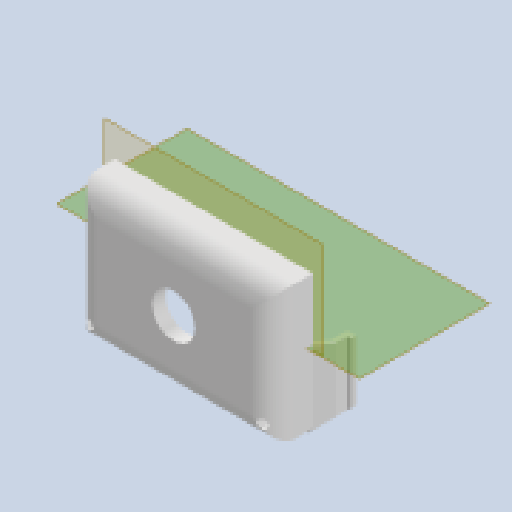
# Autodesk Inventor part: крышка камера
Saved by Autodesk Inventor 2024.2 (Build 282272000, 272)
## iProperties
Created: 2025-10-05
Part Number: крышка камера
Material: Типовые
Document SubType Name: Modeling
Designer: katya_notebook
Density: 1 g/cm^3
Appearance: По умолчанию
Author: katya_notebook
Autodesk Inventor part; units mm, degrees
ref_plane "YZ Plane" through (0, 0, 0) normal (1, 0, 0) x (0, 1, 0)
ref_plane "XZ Plane" through (0, 0, 0) normal (0, 1, 0) x (-1, 0, 0)
ref_plane "XY Plane" through (0, 0, 0) normal (0, 0, 1) x (1, 0, 0)
ref_plane "РабПлоскость1" through (0, 0, 0) normal (0, 0, 1) x (1, 0, 0)
sketch "Эскиз1" plane through (0, 0, 0) normal (0, 0, 1) x (1, 0, 0)
  line L0 (73.8991, -26.68) -> (-0.5009, -26.68) projected
  line L1 (53.6991, 17.5343) -> (19.6991, 17.5343) projected
  line L2 (0, 17.5343) -> (0, -26.68)
  line L3 (0, -26.68) -> (73.3991, -26.68)
  line L4 (73.3991, -13.5) -> (73.3991, 13.5) projected
  line L5 (73.3991, 17.5343) -> (73.3991, -26.68)
  line L6 (0, 17.5343) -> (0, 23.0229)
  line L7 (73.3991, 17.5343) -> (73.3991, 23.0229)
  line L8 (73.3991, 23.0229) -> (0, 23.0229)
  constraints: 12 end point, 3 perpendicular, 1 horizontal, 1 point on line, 1 vertical
extrude "Выдавливание1" add sketch "Эскиз1" along normal blind 15
sketch "Эскиз2" plane through (0, 0, 0) normal (0, 0, -1) x (-1, 0, 0)
  point P0 (0, 0)
sketch "Эскиз3" plane through (0, 0, 0) normal (0, 0, 1) x (1, 0, 0)
  circle A0 centre (36.6991, -1.4657) radius 8 projected
  line L0 (53.6991, 17.5343) -> (19.6991, 17.5343) projected
  line L1 (19.6991, -20.4657) -> (53.6991, -20.4657) projected
  line L2 (17.6991, 15.5343) -> (17.6991, -18.4657) projected
  line L3 (55.6991, -18.4657) -> (55.6991, 15.5343) projected
  line L4 (57.6991, 19.5343) -> (15.6991, 19.5343)
  line L5 (15.6991, 19.5343) -> (15.6991, -22.4657)
  line L6 (15.6991, -22.4657) -> (57.6991, -22.4657)
  line L7 (57.6991, -22.4657) -> (57.6991, 19.5343)
  line L8 (57.6991, 19.5343) -> (15.6991, -22.4657) construction
  line L9 (15.6991, 19.5343) -> (57.6991, -22.4657) construction
  point P0 (0, 0)
  dimension "d2" = 42
  dimension "d3" = 42
  constraints: 12 end point, 2 midpoint, 2 parallel, 1 horizontal, 1 perpendicular
  measures "d2" distance of L6.end L5.end
  measures "d3" distance of L4.start L6.end
extrude "Выдавливание2" cut sketch "Эскиз3" along normal blind 15
sketch "Эскиз4" plane through (36.6991, -1.4657, 15) normal (0, 0, 1) x (1, 0, 0)
  circle A0 centre (0, 0) radius 8
  point P0 (-36.6991, 1.4657)
  dimension "d8" = 16
  constraints: 1 centre point
  measures "d8" diameter of A0
extrude "Выдавливание3" cut sketch "Эскиз4" against normal blind 15
sketch "Эскиз5" plane through (0, 0, 15) normal (0, 0, 1) x (1, 0, 0)
  line L0 (15.6991, 19.5343) -> (57.6991, 19.5343) projected
  line L1 (15.6991, -22.4657) -> (15.6991, 19.5343) projected
  line L2 (15.6991, 19.5343) -> (57.6991, 19.5343)
  line L3 (57.6991, 19.5343) -> (57.6991, -22.4657)
  line L4 (57.6991, -22.4657) -> (15.6991, -22.4657)
  line L5 (15.6991, -22.4657) -> (15.6991, 19.5343)
  circle A0 centre (36.6991, -1.4657) radius 8 projected
  circle A1 centre (36.6991, -1.4657) radius 8
  point P0 (0, 0)
  constraints: 8 end point, 2 parallel, 1 centre point, 1 coincident, 1 concentric, 1 horizontal, 1 perpendicular
extrude "Выдавливание4" add sketch "Эскиз5" against normal blind 5
sketch "Эскиз6" plane through (0, 0, 15) normal (0, 0, 1) x (1, 0, 0)
  circle A0 centre (4.8591, -20.5207) radius 1.7 projected
  circle A1 centre (68.6491, -20.5207) radius 1.7 projected
  point P0 (0, 0)
extrude "Выдавливание5" cut sketch "Эскиз6" against normal blind 15
ref_plane "РабПлоскость2" through (83.2991, 0, -26.4849) normal (0, -1, 0) x (-1, 0, 0)
sketch "Эскиз7" plane through (83.2991, 0, -26.4849) normal (0, -1, 0) x (-1, 0, 0)
  line L0 (86.92, -21.6571) -> (83.2991, -26.4849) projected
  line L1 (86.92, -17.4429) -> (86.92, -21.6571) projected
  line L2 (91.12, -17.4429) -> (86.92, -17.4429) projected
  line L3 (83.2991, -26.4849) -> (86.92, -21.6571)
  line L4 (86.92, -21.6571) -> (86.92, -17.4429)
  line L5 (88.2462, -17.4429) -> (86.92, -17.4429)
  line L6 (88.2462, -17.4429) -> (88.2462, -15.4429)
  line L7 (88.2462, -15.4429) -> (87.1096, -15.4429)
  line L8 (87.1096, -15.4429) -> (85.1096, -15.4429)
  line L9 (83.2991, -26.4849) -> (81.2991, -26.4849)
  line L10 (9.9, -26.4849) -> (83.2991, -26.4849) projected
  line L11 (84.92, -21.6571) -> (84.92, -15.4429)
  line L12 (84.92, -15.4429) -> (85.1096, -15.4429)
  line L13 (84.92, -21.6571) -> (81.2991, -26.4849)
  line L14 (46.6, -4.8277) -> (46.6, -53.2548)
  line L15 (6.28, -21.6571) -> (9.9009, -26.4849)
  line L16 (6.28, -17.4429) -> (6.28, -21.6571)
  line L17 (9.9009, -26.4849) -> (6.28, -21.6571)
  line L18 (6.28, -21.6571) -> (6.28, -17.4429)
  line L19 (4.9538, -17.4429) -> (6.28, -17.4429)
  line L20 (4.9538, -17.4429) -> (4.9538, -15.4429)
  line L21 (4.9538, -15.4429) -> (6.0904, -15.4429)
  line L22 (6.0904, -15.4429) -> (8.0904, -15.4429)
  line L23 (9.9009, -26.4849) -> (11.9009, -26.4849)
  line L24 (8.28, -21.6571) -> (8.28, -15.4429)
  line L25 (8.28, -15.4429) -> (8.0904, -15.4429)
  line L26 (8.28, -21.6571) -> (11.9009, -26.4849)
  dimension "d13" = 2
  dimension "d14" = 2
  dimension "d15" = 2
  dimension "d16" = 2
  constraints: 46 end point, 10 symmetric about line, 3 vertical, 2 collinear, 2 horizontal, 2 perpendicular, 2 point on line
  measures "d13" distance of L6.end L5.start
  measures "d14" distance of L8.end L7.end
  measures "d15" distance of L0.end L9.end
  measures "d16" distance of L11.start L0.start
ref_plane "РабПлоскость3" through (-3.0009, -24.18, -16.4278) normal (0.7071068, 0.7071068, 0) x (-0.7071068, 0.7071068, 0)
extrude "Выдавливание6" add sketch "Эскиз7" along normal up to surface contours L0 L9 L13 L11 L12 L8 L7 L6 L2 L1 surface through (-3.0009, -24.18, -16.4278) normal (0.7071068, 0.7071068, 0)
ref_plane "РабПлоскость4" through (83.2991, 0, -26.4849) normal (0, -1, 0) x (-1, 0, 0)
sketch "Эскиз8" plane through (83.2991, 0, -26.4849) normal (0, -1, 0) x (-1, 0, 0)
  line L0 (6.28, -17.4429) -> (6.28, -21.6571) projected
  line L1 (6.28, -21.6571) -> (9.295, -25.6771) projected
  line L2 (6.28, -21.6571) -> (9.9009, -26.4849)
  line L3 (9.9009, -26.4849) -> (11.8856, -26.4849)
  line L4 (9.9, -26.4849) -> (83.2991, -26.4849) projected
  line L5 (6.28, -17.4429) -> (6.28, -21.6571)
  line L6 (8.28, -21.6571) -> (11.9009, -26.4849) projected
  line L7 (11.9009, -26.4849) -> (8.28, -21.6571)
  line L8 (8.28, -21.6571) -> (8.28, -15.4429)
  line L9 (4.9538, -17.4429) -> (6.28, -17.4429) projected
  line L10 (3.08, -17.4429) -> (6.28, -17.4429) projected
  line L11 (4.9538, -17.4429) -> (4.9538, -15.4429) projected
  line L12 (4.9538, -15.4429) -> (6.0904, -15.4429) projected
  line L13 (4.9538, -17.4429) -> (4.9538, -15.4429)
  line L14 (8.28, -21.6571) -> (8.28, -15.4429) projected
  line L15 (4.9538, -15.4429) -> (8.28, -15.4429)
  line L16 (4.9538, -17.4429) -> (6.28, -17.4429)
  constraints: 16 end point, 2 point on line, 2 vertical, 1 collinear, 1 horizontal, 1 perpendicular
ref_plane "РабПлоскость5" through (73.8991, -26.68, -16.4278) normal (-0.7071068, 0.7071068, 0) x (0, 0, 1)
extrude "Выдавливание7" add sketch "Эскиз8" along normal up to surface surface through (73.8991, -26.68, -16.4278) normal (-0.7071068, 0.7071068, 0)
fillet "Сопряжение2" radius 8 4 edges at (0, -1.8286, 15) (36.6996, 23.0229, 15) (36.6996, -26.68, 15) (73.3991, -1.8286, 15)
